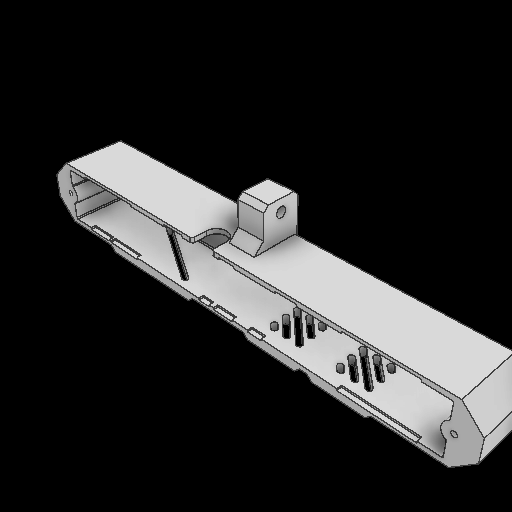
# Autodesk Inventor part: DepthCameraHousing
Saved by Autodesk Inventor 2025.2 (Build 292293000, 293)
## iProperties
Created: 2026-02-04
Part Number: DepthCameraHousing
Material: Generic
Document SubType Name: Modeling
Designer: valer
Density: 1 g/cm^3
Appearance: Default
Author: valer
Autodesk Inventor part; units mm, degrees
ref_plane "YZ Plane" through (0, 0, 0) normal (1, 0, 0) x (0, 1, 0)
ref_plane "XZ Plane" through (0, 0, 0) normal (0, 1, 0) x (-1, 0, 0)
ref_plane "XY Plane" through (0, 0, 0) normal (0, 0, 1) x (1, 0, 0)
sketch "Base" plane through (0, 0, 0) normal (0, 0, 1) x (1, 0, 0)
  line L0 (-81.75, 10.35) -> (81.75, 10.35)
  line L1 (81.75, 10.35) -> (81.75, -10.35)
  line L2 (81.75, -10.35) -> (-81.75, -10.35)
  line L3 (-81.75, -10.35) -> (-81.75, 10.35)
  line L4 (-81.75, 10.35) -> (81.75, -10.35) construction
  line L5 (81.75, 10.35) -> (-81.75, -10.35) construction
  line L6 (-122.5, 0) -> (122.5, 0) construction
  line L7 (0, -17.29) -> (0, 17.29) construction
  line L8 (83.75, 12.35) -> (-83.75, 12.35)
  line L9 (-83.75, 12.35) -> (-83.75, -12.35)
  line L10 (-83.75, -12.35) -> (83.75, -12.35)
  line L11 (83.75, -12.35) -> (83.75, 12.35)
  circle A0 centre (-83.5, 0) radius 4
  circle A1 centre (83.5, 0) radius 4
  line L12 (-83.5, 0) -> (83.5, 0) construction
  circle A2 centre (-83.5, 0) radius 1
  circle A3 centre (83.5, 0) radius 1
  point P0 (0, 0)
  point P1 (-83.75, 3.9922)
  point P2 (-83.75, -3.9922)
  point P3 (83.75, -3.9922)
  point P4 (83.75, 3.9922)
  point P5 (-81.75, 3.5969)
  point P6 (81.75, 3.5969)
  point P7 (81.75, -3.5969)
  point P8 (-81.75, -3.5969)
  dimension "d0" = 20.7
  dimension "d14" = 2
  dimension "d51" = 8
  dimension "d52" = 167
  dimension "d53" = 163.5
  dimension "d54" = 2
  dimension "d55" = 2
  constraints: 22 end point, 4 centre point, 4 parallel, 3 midpoint, 2 coincident, 2 perpendicular, 2 point on line, 1 collinear, 1 equal radius, 1 horizontal, 3 other
  measures "d0" distance between parallel lines of L2 L0
  measures "d14" distance between parallel lines of L0 L8
  measures "d51" diameter of A0
  measures "d52" distance of L12.end L12.start
  measures "d53" distance between parallel lines of L1 L3
  measures "d54" diameter of A2
  measures "d55" diameter of A3
extrude "BaseFeature" add sketch "Base" along normal blind 22.5 contours L3 A0 L9 L8 L11 A1 L1 L0 | A0 L3 | L3 A0 L9 A2 | A1 L11 A3 L1 | L1 A1 | L3 L2 L1 A1 L11 L10 L9 A0 | L9 A2 A0 | A1 L11 A3
extrude "BackFeature" add sketch "Base" against normal blind 3 contours L3 A0 L9 L8 L11 A1 L1 L0 | L0 L1 A1 L2 L3 A0 | A0 L3 | L3 A0 L9 A2 | A1 L11 A3 L1 | L1 A1 | L3 L2 L1 A1 L11 L10 L9 A0 | L9 A2 A0 | A1 L11 A3
sketch "Mount" plane through (0, 0, -3) normal (0, 0, -1) x (-1, 0, 0)
  line L0 (126, 0) -> (-126, 0) construction
  line L1 (0, -19.25) -> (0, 19.25) construction
  line L2 (83.75, 12.35) -> (-83.75, 12.35) projected
  line L3 (5.5, 12.35) -> (2.5, 12.35)
  line L4 (5.5, 28.35) -> (5.5, 12.35)
  line L5 (-5.5, 28.35) -> (-5.5, 12.35)
  line L6 (5.5, 28.35) -> (-5.5, 28.35)
  point P0 (0, 0)
  point P1 (-5.5, 12.35)
  dimension "d70" = 16
  dimension "d121" = 11
  constraints: 12 end point, 3 horizontal, 2 symmetric about line, 1 point on line, 1 vertical, 4 other
  measures "d70" distance of L4.start L3.start
  measures "d121" distance between parallel lines of L5 L4
extrude "MountFeature" add sketch "Mount" against normal blind 15
chamfer "MountChamferFeature" distance 2 angle 45 2 edges at (0, 28.35, -3) (0, 28.35, 12)
sketch "Sides" plane through (0, 0, -3) normal (0, 0, -1) x (-1, 0, 0)
  line L0 (0, -20.568) -> (0, 36.503) construction
  line L1 (-83.75, -12.35) -> (83.75, -12.35) projected
  line L2 (-83.75, -12.35) -> (-91.5, -4.6)
  line L3 (128.1, 0) -> (-128.1, 0) construction
  line L4 (-91.5, -4.6) -> (-91.5, 0)
  arc A0 (-77.585, 12.415) -> (-77.585, -12.415) centre (-77.585, 0) ccw construction
  arc A1 (-83.75, 3.9922) -> (-83.75, -3.9922) centre (-83.5, 0) ccw projected
  line L5 (83.75, -12.35) -> (91.5, -4.6)
  line L6 (91.5, -4.6) -> (91.5, 0)
  line L7 (-83.75, 12.35) -> (-91.5, 4.6)
  line L8 (-91.5, 4.6) -> (-91.5, 0)
  line L9 (83.75, 12.35) -> (91.5, 4.6)
  line L10 (91.5, 4.6) -> (91.5, 0)
  line L11 (83.75, -12.35) -> (83.75, -3.9922) projected
  arc A2 (83.75, -3.9922) -> (83.75, 3.9922) centre (83.5, 0) ccw projected
  line L12 (83.75, 3.9922) -> (83.75, 12.35) projected
  line L13 (-83.75, -3.9922) -> (-83.75, -12.35) projected
  line L14 (-83.75, 12.35) -> (-83.75, 3.9922) projected
  point P0 (0, 0)
  point P1 (-87.5, 0)
  dimension "d76" = 4
  dimension "d77" = 45
  constraints: 16 end point, 6 symmetric about line, 1 perpendicular, 1 point on circle, 1 point on line
  measures "d76" distance of L4.end point (-87.5, 0)
  measures "d77" angle of L2 L3
extrude "SidesFeature" add sketch "Sides" against normal up to surface (25.5 mm away)
sketch "Decorative" plane through (0, 0, 22.5) normal (0, 0, 1) x (1, 0, 0)
  line L0 (-83.75, -12.35) -> (83.75, -12.35) projected
  line L1 (58, -12.35) -> (56, -14.35)
  line L2 (56, -14.35) -> (36, -14.35)
  line L3 (36, -14.35) -> (34, -12.35)
  circle A0 centre (46, 0) radius 9.875 construction
  line L4 (46, -14.35) -> (46, 0) construction
  circle A1 centre (19, 0) radius 9.875 construction
  line L5 (31, -12.35) -> (29, -14.35)
  line L6 (29, -14.35) -> (9, -14.35)
  line L7 (9, -14.35) -> (7, -12.35)
  line L8 (19, -14.35) -> (19, 0) construction
  line L9 (-17, -12.35) -> (-19, -14.35)
  line L10 (-19, -14.35) -> (-59, -14.35)
  line L11 (-59, -14.35) -> (-61, -12.35)
  point P0 (0, 0)
  dimension "d80" = 45
  dimension "d81" = 45
  dimension "d82" = 2
  dimension "d83" = 20
  dimension "d84" = 45
  dimension "d85" = 45
  dimension "d86" = 40
  dimension "d89" = 45
  dimension "d90" = 45
  dimension "d91" = 24
  constraints: 22 end point, 6 point on line, 3 collinear, 2 midpoint, 2 perpendicular, 1 horizontal, 1 parallel, 1 vertical
  measures "d80" angle of L0 L3
  measures "d81" angle of L0 L1
  measures "d82" distance between parallel lines of L0 L2
  measures "d83" distance of L1.end L2.end
  measures "d84" angle of L0 L5
  measures "d85" angle of L0 L7
  measures "d86" distance of L9.end L10.end
  measures "d89" angle of L0 L9
  measures "d90" angle of L0 L11
  measures "d91" distance of L9.start L7.end
extrude "DecorativeFeature" add sketch "Decorative" against normal up to surface (25.5 mm away)
chamfer "BackChamferFeature" distance 1 angle 45 21 edges at (-72.375, -12.35, -3) (-87.625, -8.475, -3) (-91.5, 0, -3) (-87.625, 8.475, -3) (-44.625, 12.35, -3) (-60, -13.35, -3) (-39, -14.35, -3) (-18, -13.35, -3) (-5, -12.35, -3) (8, -13.35, -3) (19, -14.35, -3) (30, -13.35, -3) (32.5, -12.35, -3) (35, -13.35, -3) (46, -14.35, -3) (57, -13.35, -3) (70.875, -12.35, -3) (87.625, -8.475, -3) (91.5, 0, -3) (87.625, 8.475, -3) (44.625, 12.35, -3)
sketch "MountHole" plane through (5.5, 12.35, 12) normal (1, 0, 0) x (0, 0, -1)
  line L0 (13, 16) -> (2, 16) projected
  line L1 (7.5, 16) -> (7.5, 11) construction
  circle A0 centre (7.5, 11) radius 2
  point P0 (12, -12.35)
  point P1 (15, 16)
  point P2 (0, 16)
  dimension "d97" = 4
  dimension "d98" = 5
  constraints: 2 end point, 1 centre point, 1 coincident, 1 midpoint, 1 vertical
  measures "d97" diameter of A0
  measures "d98" distance of L1.start L1.end
extrude "MountHoleFeature" cut sketch "MountHole" along normal through all both and the other way through all
sketch "DecorativeHoles" plane through (36, -14.35, 22.5) normal (0, -1, 0) x (1, 0, 0)
  line L0 (20, -24.5) -> (0, -24.5) construction
  line L1 (20, 0) -> (20, -24.5) construction
  line L2 (0, 0) -> (20, 0) construction
  line L3 (0, 0) -> (0, -24.5) construction
  line L4 (-7, -24.5) -> (-27, -24.5) construction
  line L5 (-7, 0) -> (-7, -24.5) construction
  line L6 (-27, 0) -> (-7, 0) construction
  line L7 (-27, 0) -> (-27, -24.5) construction
  line L8 (-55, -24.5) -> (-95, -24.5) construction
  line L9 (-55, 0) -> (-55, -24.5) construction
  line L10 (-95, 0) -> (-55, 0) construction
  line L11 (-95, 0) -> (-95, -24.5) construction
  line L12 (16, -6.5) -> (4, -18.5) construction
  line L13 (15.1868, -5.6868) -> (3.1868, -17.6868)
  line L14 (4.8132, -19.3132) -> (16.8132, -7.3132)
  arc A0 (16.8132, -7.3132) -> (15.1868, -5.6868) centre (16, -6.5) ccw
  arc A1 (3.1868, -17.6868) -> (4.8132, -19.3132) centre (4, -18.5) ccw
  line L15 (20, -18.5) -> (0, -18.5) construction
  line L16 (20, -4) -> (0, -4) construction
  line L17 (14.5858, -18.5) -> (16, -17.0858) construction
  line L18 (13.7726, -17.6868) -> (15.1868, -16.2726)
  line L19 (16.8132, -17.899) -> (15.399, -19.3132)
  arc A2 (13.7726, -17.6868) -> (15.399, -19.3132) centre (14.5858, -18.5) ccw
  arc A3 (16.8132, -17.899) -> (15.1868, -16.2726) centre (16, -17.0858) ccw
  line L20 (4, -7.9142) -> (5.4142, -6.5) construction
  line L21 (4.8132, -8.7274) -> (6.2274, -7.3132)
  line L22 (4.601, -5.6868) -> (3.1868, -7.101)
  arc A4 (3.1868, -7.101) -> (4.8132, -8.7274) centre (4, -7.9142) ccw
  arc A5 (6.2274, -7.3132) -> (4.601, -5.6868) centre (5.4142, -6.5) ccw
  line L23 (9.2929, -18.5) -> (16, -11.7929) construction
  line L24 (10.1061, -19.3132) -> (16.8132, -12.6061)
  line L25 (15.1868, -10.9797) -> (8.4797, -17.6868)
  arc A6 (8.4797, -17.6868) -> (10.1061, -19.3132) centre (9.2929, -18.5) ccw
  arc A7 (16.8132, -12.6061) -> (15.1868, -10.9797) centre (16, -11.7929) ccw
  line L26 (4, -13.2071) -> (10.7071, -6.5) construction
  line L27 (3.1868, -12.3939) -> (9.8939, -5.6868)
  line L28 (11.5203, -7.3132) -> (4.8132, -14.0203)
  arc A8 (3.1868, -12.3939) -> (4.8132, -14.0203) centre (4, -13.2071) ccw
  arc A9 (11.5203, -7.3132) -> (9.8939, -5.6868) centre (10.7071, -6.5) ccw
  line L29 (20, -18.5) -> (0, -4) construction
  line L30 (-2, -24.5) -> (-5, -24.5) projected
  line L31 (-5, 0) -> (-2, 0) projected
  line L32 (-10.1868, -17.899) -> (-11.601, -19.3132)
  arc A10 (-13.2274, -17.6868) -> (-11.601, -19.3132) centre (-12.4142, -18.5) ccw
  arc A11 (-10.1868, -17.899) -> (-11.8132, -16.2726) centre (-11, -17.0858) ccw
  line L33 (-13.2274, -17.6868) -> (-11.8132, -16.2726)
  line L34 (-16.8939, -19.3132) -> (-10.1868, -12.6061)
  arc A12 (-18.5203, -17.6868) -> (-16.8939, -19.3132) centre (-17.7071, -18.5) ccw
  line L35 (-11.8132, -10.9797) -> (-18.5203, -17.6868)
  arc A13 (-10.1868, -12.6061) -> (-11.8132, -10.9797) centre (-11, -11.7929) ccw
  line L36 (-22.1868, -19.3132) -> (-10.1868, -7.3132)
  arc A14 (-10.1868, -7.3132) -> (-11.8132, -5.6868) centre (-11, -6.5) ccw
  line L37 (-11.8132, -5.6868) -> (-23.8132, -17.6868)
  arc A15 (-23.8132, -17.6868) -> (-22.1868, -19.3132) centre (-23, -18.5) ccw
  arc A16 (-23.8132, -12.3939) -> (-22.1868, -14.0203) centre (-23, -13.2071) ccw
  line L38 (-15.4797, -7.3132) -> (-22.1868, -14.0203)
  line L39 (-23.8132, -12.3939) -> (-17.1061, -5.6868)
  arc A17 (-15.4797, -7.3132) -> (-17.1061, -5.6868) centre (-16.2929, -6.5) ccw
  arc A18 (-20.7726, -7.3132) -> (-22.399, -5.6868) centre (-21.5858, -6.5) ccw
  line L40 (-22.1868, -8.7274) -> (-20.7726, -7.3132)
  line L41 (-22.399, -5.6868) -> (-23.8132, -7.101)
  arc A19 (-23.8132, -7.101) -> (-22.1868, -8.7274) centre (-23, -7.9142) ccw
  point P0 (-36, -22.5)
  point P1 (10, -12.5)
  point P2 (15.2929, -17.7929)
  point P3 (12.6464, -15.1464)
  point P4 (4.7071, -7.2071)
  dimension "d102" = 45
  dimension "d104" = 4
  dimension "d105" = 4
  dimension "d106" = 4
  dimension "d107" = 4
  dimension "d108" = 3.7426
  dimension "d109" = 3.7426
  dimension "d110" = 3.7426
  dimension "d111" = 3.7426
  dimension "d113" = 4
  dimension "d114" = 4
  dimension "d115" = 4
  dimension "d118" = 6
  dimension "d119" = 2
  dimension "d120" = 1.15
  dimension "d124" = 27
  constraints: 66 end point, 40 point on circle, 20 centre point, 12 symmetric about line, 12 tangent, 7 point on line, 5 parallel, 4 midpoint, 2 equal radius, 2 perpendicular, 1 horizontal, 54 other
  measures "d102" angle of L12 L1
  measures "d104" distance from line of L1 L12.start
  measures "d105" distance between parallel lines of L2 L16
  measures "d106" distance from line of L1 L17.end
  measures "d107" distance from line of L1 L23.end
  measures "d108" distance between parallel lines of L23 L17
  measures "d109" distance between parallel lines of L12 L23
  measures "d110" distance between parallel lines of L26 L12
  measures "d111" distance from line of point (4.707, -7.207) L26
  measures "d113" distance from line of L3 L20.start
  measures "d114" distance from line of L3 L12.end
  measures "d115" distance from line of L3 L26.start
  measures "d118" distance between parallel lines of L0 L15
  measures "d119" distance of L17.start L17.end
  measures "d120" radius of A1
  measures "d124" distance of L19.start L32.start
extrude "DecorativeHolesFeature" cut sketch "DecorativeHoles" against normal up to surface (4 mm away)
sketch "OneMoreDecorativeHole" plane through (-59, -14.35, 22.5) normal (0, -1, 0) x (1, 0, 0)
  line L0 (34, -4) -> (6, -20.5) construction
  line L1 (33.4162, -3.0092) -> (5.4162, -19.5092)
  line L2 (6.5838, -21.4908) -> (34.5838, -4.9908)
  arc A0 (34.5838, -4.9908) -> (33.4162, -3.0092) centre (34, -4) ccw
  arc A1 (5.4162, -19.5092) -> (6.5838, -21.4908) centre (6, -20.5) ccw
  arc A2 (71.1868, -17.6868) -> (72.8132, -19.3132) centre (72, -18.5) ccw projected
  line L3 (0, 0) -> (40, 0) projected
  line L4 (40, 0) -> (40, -24.5) projected
  line L5 (0, 0) -> (0, -24.5) projected
  line L6 (40, -24.5) -> (0, -24.5) projected
  point P0 (59, -22.5)
  point P1 (20, -12.25)
  dimension "d132" = 4
  dimension "d133" = 6
  dimension "d134" = 6
  dimension "d135" = 4
  constraints: 8 end point, 4 point on circle, 4 tangent, 2 centre point, 1 equal radius, 1 midpoint, 1 parallel
  measures "d132" distance from line of L3 L0.start
  measures "d133" distance from line of L4 L0.start
  measures "d134" distance from line of L5 L0.end
  measures "d135" distance from line of L6 L0.end
chamfer "FrontChamferFeature" distance 4 angle 45 1 edges at (0, 12.35, 12)
extrude "OneMoreDecorativeHoleFeature" cut sketch "OneMoreDecorativeHole" against normal up to surface (4 mm away) contours A0 L2 A1 L1
fillet "InsideFilletsFeature" radius 0.5 16 edges at (81.75, -10.35, 11.25) (81.75, -3.5969, 11.25) (81.75, 3.5969, 11.25) (81.75, 10.35, 11.25) (0, 10.35, 0) (81.75, 6.9734, 0) (79.5, 0, 0) (81.75, -6.9734, 0) (0, -10.35, 0) (-81.75, -6.9734, 0) (-79.5, 0, 0) (-81.75, -3.5969, 11.25) (-81.75, 3.5969, 11.25) (-81.75, 6.9734, 0) (-81.75, 10.35, 11.25) (-81.75, -10.35, 11.25)
sketch "CableHole" plane through (-83.75, 12.35, 22.5) normal (0, 1, 0) x (1, 0, 0)
  line L0 (66.75, 0) -> (90.75, 0) projected
  line L1 (77.25, 0) -> (68.25, 0)
  line L2 (68.25, 0) -> (68.25, 6)
  line L3 (68.25, 6) -> (77.25, 6) construction
  line L4 (77.25, 6) -> (77.25, 0)
  circle A0 centre (72.75, 6) radius 4.5
  line L5 (78.25, 10.5) -> (78.25, 6.5) projected
  line L6 (78.25, 10.5) -> (89.25, 10.5) projected
  point P0 (83.75, 22.5)
  point P1 (68.25, 6)
  point P2 (68.25, 0)
  dimension "d179" = 9
  dimension "d180" = 1
  constraints: 8 end point, 2 parallel, 2 tangent, 1 centre point, 1 coincident, 1 horizontal, 1 midpoint, 1 perpendicular, 1 point on line
  measures "d179" distance between parallel lines of L2 L4
  measures "d180" distance between parallel lines of L5 L4
extrude "CableHoleFeature" cut sketch "CableHole" against normal up to surface (2 mm away)
fillet "CableHoleFilletsFeature" radius 1 2 edges at (-6.5, 11.35, 22.5) (-15.5, 11.35, 22.5)
sketch "SnapFitHolesBottom" plane through (5.5, 10.35, -2) normal (0, 1, 0) x (1, 0, 0)
  line L0 (75.75, -24.5) -> (-86.75, -24.5) projected
  line L1 (66.45, -24.5) -> (39.95, -24.5)
  line L2 (39.95, -24.5) -> (39.95, -22.5)
  line L3 (39.95, -22.5) -> (66.45, -22.5)
  line L4 (66.45, -22.5) -> (66.45, -24.5)
  line L5 (-11, -24.5) -> (75.75, -24.5) projected
  line L6 (23.45, -24.5) -> (14.95, -24.5)
  line L7 (14.95, -24.5) -> (14.95, -22.5)
  line L8 (14.95, -22.5) -> (23.45, -22.5)
  line L9 (23.45, -22.5) -> (23.45, -24.5)
  line L10 (-2.4236, -24.5) -> (-8.9236, -24.5)
  line L11 (-8.9236, -24.5) -> (-8.9236, -22.5)
  line L12 (-8.9236, -22.5) -> (-2.4236, -22.5)
  line L13 (-2.4236, -22.5) -> (-2.4236, -24.5)
  line L14 (-26, -24.5) -> (-35, -24.5)
  line L15 (-35, -24.5) -> (-35, -22.5)
  line L16 (-35, -22.5) -> (-26, -22.5)
  line L17 (-26, -22.5) -> (-26, -24.5)
  line L18 (-52, -24.5) -> (-78, -24.5)
  line L19 (-78, -24.5) -> (-78, -22.5)
  line L20 (-78, -22.5) -> (-52, -22.5)
  line L21 (-52, -22.5) -> (-52, -24.5)
  line L22 (-5.5, 6.1) -> (-5.5, -29.6) construction
  point P0 (-5.5, -2)
  point P1 (-5.5, -24.5)
  point P2 (19.2, -22.5)
  point P3 (53.2, -22.5)
  point P4 (-30.5, -22.5)
  point P5 (-65, -22.5)
  dimension "d202" = 26.5
  dimension "d203" = 8.5
  dimension "d204" = 6.5
  dimension "d205" = 9
  dimension "d206" = 26
  dimension "d207" = 2
  dimension "d208" = 24.7
  dimension "d209" = 34
  dimension "d210" = 25
  dimension "d211" = 59.5
  constraints: 40 end point, 10 parallel, 6 point on line, 5 horizontal, 5 midpoint, 5 perpendicular, 4 collinear
  measures "d202" distance of L2.end L3.end
  measures "d203" distance of L7.end L8.end
  measures "d204" distance of L11.end L12.end
  measures "d205" distance of L15.end L16.end
  measures "d206" distance of L19.end L20.end
  measures "d207" distance of L3.end L1.start
  measures "d208" distance from line of point (19.2, -22.5) L22
  measures "d209" distance of point (53.2, -22.5) point (19.2, -22.5)
  measures "d210" distance from line of point (-30.5, -22.5) L22
  measures "d211" distance from line of L22 point (-65, -22.5)
sketch "SnapFitHolesTop" plane through (-59, -10.35, 22.5) normal (0, -1, 0) x (1, 0, 0)
  line L0 (140.25, 0) -> (-22.25, 0) projected
  line L1 (-14, 0) -> (-3, 0)
  line L2 (-3, 0) -> (-3, -2)
  line L3 (-3, -2) -> (-14, -2)
  line L4 (-14, -2) -> (-14, 0)
  line L5 (12.85, 0) -> (-2, 0)
  line L6 (-2, 0) -> (-2, -2)
  line L7 (-2, -2) -> (12.85, -2)
  line L8 (12.85, -2) -> (12.85, 0)
  line L9 (45.35, 0) -> (50.35, 0)
  line L10 (50.35, 0) -> (50.35, -2)
  line L11 (50.35, -2) -> (45.35, -2)
  line L12 (45.35, -2) -> (45.35, 0)
  line L13 (52.35, 0) -> (61, 0)
  line L14 (61, 0) -> (61, -2)
  line L15 (61, -2) -> (52.35, -2)
  line L16 (52.35, -2) -> (52.35, 0)
  line L17 (68, 0) -> (68, -24.5) projected
  line L18 (68, 0) -> (74, 0)
  line L19 (74, 0) -> (74, -2)
  line L20 (74, -2) -> (68, -2)
  line L21 (68, -2) -> (68, 0)
  line L22 (104.5, 0) -> (132.5, 0)
  line L23 (132.5, 0) -> (132.5, -2)
  line L24 (132.5, -2) -> (104.5, -2)
  line L25 (104.5, -2) -> (104.5, 0)
  line L26 (59, -30.6) -> (59, 5.1) construction
  line L27 (-2, -24.5) -> (-2, 0) projected
  point P0 (59, -22.5)
  point P1 (-3, 0)
  point P2 (68, -2)
  point P3 (74, 0)
  dimension "d212" = 2
  dimension "d213" = 2
  dimension "d214" = 6
  dimension "d215" = 28
  dimension "d216" = 30.5
  dimension "d217" = 2
  dimension "d218" = 5
  dimension "d219" = 8.65
  dimension "d220" = 32.5
  dimension "d221" = 1
  dimension "d222" = 11
  constraints: 48 end point, 12 parallel, 6 collinear, 6 horizontal, 6 perpendicular, 6 other
  measures "d212" distance of L3.end L1.start
  measures "d213" distance from line of L14.end L26
  measures "d214" distance of L19.end L20.end
  measures "d215" distance of L23.end L24.end
  measures "d216" distance of L24.end L19.end
  measures "d217" distance of L15.end L10.end
  measures "d218" distance of L10.end L11.end
  measures "d219" distance from line of L26 L10.end
  measures "d220" distance of L11.end L7.end
  measures "d221" distance of L6.end L2.end
  measures "d222" distance of L2.end L3.end
extrude "SnapFitHolesBottomFeature" cut sketch "SnapFitHolesBottom" along normal blind 0.75
extrude "SnapFitHolesTopFeature" cut sketch "SnapFitHolesTop" along normal blind 0.75
equation "\"d81\" = d80"
equation "\"d84\" = d80"
equation "\"d89\" = d80"
equation "\"d90\" = d80"
equation "\"d104\" = d103"
equation "\"d105\" = d103"
equation "\"d106\" = d103"
equation "\"d107\" = d104"
equation "\"d109\" = d108"
equation "\"d110\" = d108"
equation "\"d111\" = d108"
equation "\"d103\" = 4"
body "Solid1"
